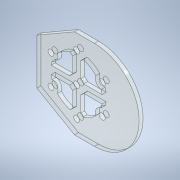
# Autodesk Inventor part: Standalone_Valve_Cover_Plate
Saved by Autodesk Inventor 2020 (Build 240168000, 168)
## iProperties
Created: 2021-07-01
Part Number: Standalone_Valve_Cover_Plate
Material: Glass
Document SubType Name: Modeling
Designer: Workshop
Density: 2.18 g/cm^3
Appearance: Clear
Author: Workshop
Autodesk Inventor part; units mm, degrees
ref_plane "YZ Plane" through (0, 0, 0) normal (1, 0, 0) x (0, 1, 0)
ref_plane "XZ Plane" through (0, 0, 0) normal (0, 1, 0) x (-1, 0, 0)
ref_plane "XY Plane" through (0, 0, 0) normal (0, 0, 1) x (1, 0, 0)
sketch "Sketch1" plane through (0, 0, 0) normal (0, 0, 1) x (1, 0, 0)
  arc A0 (-2.0132, 3.5447) -> (-3.519, 2.0549) centre (0, 0.004) ccw projected
  line L0 (-3.519, 2.0549) -> (-12.837, 2.0549) projected
  arc A1 (-12.3669, 4.0103) -> (-12.837, 2.0549) centre (-0.0002, 0.003) ccw projected
  arc A2 (-12.3669, 4.0103) -> (-9.6539, 8.7094) centre (-12.9254, 7.4655) ccw projected
  arc A3 (-3.2466, 12.5914) -> (-9.6539, 8.7094) centre (0, 0.004) ccw projected
  arc A4 (-3.2466, 12.5914) -> (-2.019, 11.4749) centre (0, 14.928) ccw projected
  line L1 (-2.019, 11.4749) -> (-2.0132, 3.5447) projected
  circle A5 centre (0, 0.002) radius 1.5 projected
  circle A6 centre (0, -14.924) radius 1.5 projected
  arc A7 (-3.519, -2.051) -> (-2.0132, -3.5408) centre (0, 0) ccw projected
  line L2 (-3.519, -2.051) -> (-12.837, -2.051) projected
  arc A8 (-12.837, -2.051) -> (-12.3669, -4.0064) centre (-0.0002, 0.0009) ccw projected
  arc A9 (-9.6539, -8.7054) -> (-12.3669, -4.0064) centre (-12.9254, -7.4615) ccw projected
  arc A10 (-9.6539, -8.7054) -> (-3.2466, -12.5874) centre (0, 0) ccw projected
  arc A11 (-2.019, -11.471) -> (-3.2466, -12.5874) centre (0, -14.924) ccw projected
  line L3 (-2.019, -11.471) -> (-2.0132, -3.5408) projected
  arc A12 (9, -22.4732) -> (8.9991, 22.4792) centre (8.9998, 0.003) ccw projected
  line L4 (8.9991, 22.4792) -> (-1.0724, 22.4758) projected
  line L5 (-1.0724, 22.4758) -> (-20, 11.548) projected
  line L6 (-20, 11.548) -> (-20, -11.546) projected
  line L7 (-20, -11.546) -> (-1.0716, -22.4743) projected
  line L8 (-1.0716, -22.4743) -> (9, -22.4732) projected
  circle A13 centre (-12.9254, 7.4635) radius 1.5 projected
  circle A14 centre (-12.9254, -7.4615) radius 1.5 projected
  circle A15 centre (0, -14.924) radius 1.5 projected
  arc A16 (3.519, 2.0549) -> (2.0132, 3.5447) centre (0, 0.004) ccw projected
  line L9 (3.519, 2.0549) -> (12.837, 2.0549) projected
  arc A17 (12.837, 2.0549) -> (12.3669, 4.0103) centre (0.0002, 0.003) ccw projected
  arc A18 (9.6539, 8.7094) -> (12.3669, 4.0103) centre (12.9254, 7.4655) ccw projected
  arc A19 (9.6539, 8.7094) -> (3.2466, 12.5914) centre (0, 0.004) ccw projected
  arc A20 (2.019, 11.4749) -> (3.2466, 12.5914) centre (0, 14.928) ccw projected
  line L10 (2.019, 11.4749) -> (2.0132, 3.5447) projected
  arc A21 (2.0132, -3.5408) -> (3.519, -2.051) centre (0, 0) ccw projected
  line L11 (3.519, -2.051) -> (12.837, -2.051) projected
  arc A22 (12.3669, -4.0064) -> (12.837, -2.051) centre (0.0002, 0.0009) ccw projected
  arc A23 (12.3669, -4.0064) -> (9.6539, -8.7054) centre (12.9254, -7.4615) ccw projected
  arc A24 (3.2466, -12.5874) -> (9.6539, -8.7054) centre (0, 0) ccw projected
  arc A25 (3.2466, -12.5874) -> (2.019, -11.471) centre (0, -14.924) ccw projected
  line L12 (2.019, -11.471) -> (2.0132, -3.5408) projected
  circle A26 centre (12.9254, -7.4615) radius 1.5 projected
  circle A27 centre (0, 14.926) radius 1.5 projected
  circle A28 centre (12.9254, 7.4635) radius 1.5 projected
  point P0 (0, 0)
extrude "Extrusion1" add sketch "Sketch1" along normal mid plane 2
body "Solid1"
